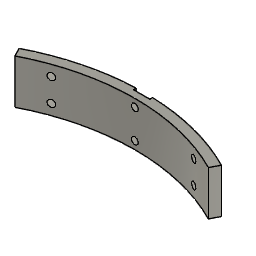
Brow Support v11 (Autodesk Fusion 360 design; units mm, degrees)
Autodesk Fusion 360 part; units mm, degrees
sketch "Curve Profile" plane through (0, 0, 0) normal (0, 0, 1) x (1, 0, 0)
  line L0 (0, 0) -> (280.8765, 0) construction
  arc A0 (100, 0) -> (0, 0) centre (50, -98.1667) ccw
  arc A1 (102.2693, 4.4554) -> (-2.2693, 4.4554) centre (50, -98.1667) ccw
  line L1 (-2.2693, 4.4554) -> (0, 0)
  line L2 (100, 0) -> (102.2693, 4.4554)
  line L3 (11.5118, 10.3783) -> (21.145, 13.7941) construction
  line L4 (50, 12) -> (50, 0) construction
  line L5 (11.5118, 10.3783) -> (13.1828, 5.6658)
  line L6 (88.4882, 10.3783) -> (86.8172, 5.6658)
  line L7 (88.4882, 10.3783) -> (78.855, 13.7941) construction
  line L8 (50, 12) -> (50, 17)
  point P0 (50, 12)
  point P1 (11.5118, 10.3783)
  point P2 (88.4882, 10.3783)
  dimension "d6" = 100
  dimension "d8" = 5
  dimension "d13" = 15
  dimension "d14" = 12
  constraint coincident L0.start A0.end
  constraint horizontal L0
  constraint coincident L0 A0.start
  constraint midpoint A0 P0
  constraint coincident A1 P1
  constraint coincident P1 L3.start
  constraint tangent A1 L3
  constraint coincident P0 L4.start
  constraint coincident L0 L4.end
  constraint perpendicular L0 L4
  constraint perpendicular L3 L5
  constraint coincident A0 L5.end
  constraint symmetric P1 L4 P2
  constraint symmetric L3.end L4 L7.end
  constraint symmetric L4 P1 P2
  constraint symmetric L4 L5.end L6.end
  constraint midpoint A1 L8.end
  constraint parallel L4 L8
  measures "d6" distance of L0.start A0.start
  measures "d13" distance of A1.end P1
  measures "d14" distance of P0 L4.end
extrude "Extrude2" add sketch "Curve Profile" along normal blind 23
ref_plane "WorkPlane4" through (11.5118, 10.3783, 0) normal (-0.334196, 0.942504, 0) x (-0.942504, -0.334196, 0)
sketch "Side Holes" plane through (11.5118, 10.3783, 0) normal (-0.334196, 0.942504, 0) x (-0.942504, -0.334196, 0)
  line L0 (0, 0) -> (0, 20.2951) construction
  circle A0 centre (0, 5.5) radius 1.75
  circle A1 centre (0, 17.5) radius 1.75
  line L1 (14.9682, 23) -> (-83.5598, 23) construction
  line L2 (0, 0) -> (-10.2209, 0) construction
  line L3 (-1.7321, 8.5) -> (-3.4641, 5.5)
  line L4 (-3.4641, 5.5) -> (-1.7321, 2.5)
  line L5 (-1.7321, 2.5) -> (1.7321, 2.5)
  line L6 (1.7321, 2.5) -> (3.4641, 5.5)
  line L7 (3.4641, 5.5) -> (1.7321, 8.5)
  line L8 (1.7321, 8.5) -> (-1.7321, 8.5)
  line L9 (-1.7321, 20.5) -> (-3.4641, 17.5)
  line L10 (-3.4641, 17.5) -> (-1.7321, 14.5)
  line L11 (-1.7321, 14.5) -> (1.7321, 14.5)
  line L12 (1.7321, 14.5) -> (3.4641, 17.5)
  line L13 (3.4641, 17.5) -> (1.7321, 20.5)
  line L14 (1.7321, 20.5) -> (-1.7321, 20.5)
  point P0 (0, 5.5)
  point P1 (0, 17.5)
  dimension "d40" = 3.5
  dimension "d41" = 3.5
  dimension "d42" = 5.5
  dimension "d43" = 5.5
  dimension "d49" = 3
  dimension "d50" = 3
  constraint coincident L0.start L2.start
  constraint vertical L0
  constraint coincident L0 P0
  constraint coincident L0 P1
  constraint coincident P0 A0.centre
  constraint horizontal L8
  constraint coincident P1 A1.centre
  constraint horizontal L14
  measures "d40" diameter of A0
  measures "d41" diameter of A1
  measures "d42" distance of P1 L1
  measures "d43" distance of P0 L2
  measures "d49" distance of P0 L8
  measures "d50" distance of P1 L14
extrude "Extrude3" cut sketch "Side Holes" against normal through all contours A0 | A1
extrude "Extrude4" cut sketch "Side Holes" against normal blind 1
ref_plane "WorkPlane5" through (50, 6, 0) normal (-1, 0, 0) x (0, -1, 0)
mirror "Mirror2" about plane through (50, 6, 0) normal (-1, 0, 0) of "Extrude3", "Extrude4"
ref_plane "WorkPlane6" through (50, 17, 0) normal (0, 1, 0) x (-1, 0, 0)
sketch "Center Holes" plane through (50, 17, 0) normal (0, 1, 0) x (-1, 0, 0)
  line L0 (0, 0) -> (0, 23) construction
  circle A0 centre (0, 4.036) radius 1.75
  line L1 (52.2693, 0) -> (-52.2693, 0)
  circle A1 centre (0, 18.964) radius 1.75
  line L2 (52.2693, 23) -> (-52.2693, 23)
  line L3 (4.25, 23) -> (-4.25, 23)
  line L4 (-4.25, 23) -> (-4.25, 0)
  line L5 (-4.25, 0) -> (4.25, 0)
  line L6 (4.25, 0) -> (4.25, 23)
  line L7 (4.25, 23) -> (-4.25, 0) construction
  line L8 (-4.25, 23) -> (4.25, 0) construction
  line L9 (0, 18.964) -> (0, 4.036)
  point P0 (0, 18.964)
  point P1 (0, 4.036)
  point P2 (0, 11.5)
  point P3 (0, 11.5)
  dimension "d54" = 3.5
  dimension "d56" = 3.5
  dimension "d64" = 8.5
  dimension "d69" = 14.928
  constraint coincident L0.start origin
  constraint vertical L0
  constraint coincident L0 P1
  constraint coincident L0 P0
  constraint coincident P0 A1.centre
  constraint coincident P1 A0.centre
  constraint midpoint L0.end L2
  constraint horizontal L3
  constraint perpendicular L3 L4
  constraint parallel L3 L5
  constraint parallel L4 L6
  constraint coincident L7 P3
  constraint coincident L8 P3
  constraint midpoint L0 P3
  constraint coincident L1 L4.end
  constraint midpoint L9 P3
  constraint coincident P3 P2
  measures "d54" diameter of A0
  measures "d56" diameter of A1
  measures "d64" distance of L4.end L5.end
  measures "d69" distance of P1 P0
extrude "Extrude5" cut sketch "Center Holes" against normal through all contours A0 | A1
extrude "Extrude7" cut sketch "Center Holes" against normal blind 1.5
equation "arc_width = 100 mm"
equation "arc_height = 12 mm"
equation "d6 = arc_width"
equation "d8 = thickness"
equation "thickness = 5 mm"
equation "depth = 23 mm"
equation "d14 = arc_height"
equation "d15 = depth"
equation "screwholed = 3.5 mm"
equation "d40 = screwholed"
equation "d41 = screwholed"
equation "d42 = d43"
equation "nut_d = 6 mm"
equation "d49 = nut_d / 2"
equation "d50 = nut_d / 2"
equation "d51 = -nut_counterbore_depth"
equation "nut_counterbore_depth = 1 mm"
equation "d54 = screwholed"
equation "d56 = screwholed"
equation "d64 = center_groove_w"
equation "center_groove_w = 8.5 mm"
equation "center_groove_depth = 1.5 mm"
equation "d67 = -center_groove_depth"
